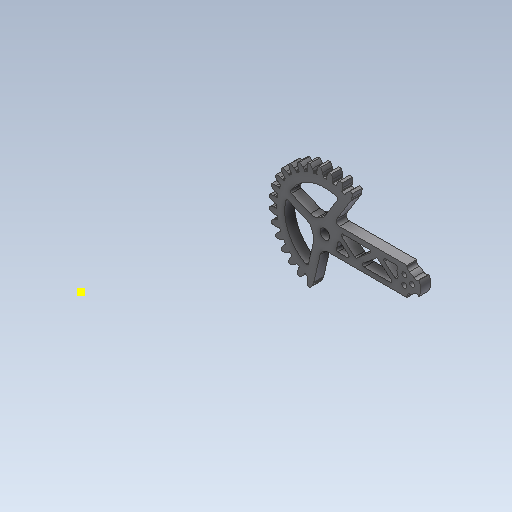
# Autodesk Inventor part: m2z32
Saved by Autodesk Inventor 2020 (Build 240168000, 168)
## iProperties
Created: 2020-01-07
Part Number: m2z32
Material: 一般
Document SubType Name: Modeling
Designer: hamaa
Density: 1 g/cm^3
Appearance: 既定
Mass: 10.1861 g
Surface Area: 77.3348 cm^2
Volume: 10.1861 cm^3
Author: hamaa
Autodesk Inventor part; units mm, degrees
(part 1 of 3)
ref_plane "YZ Plane" through (0, 0, 0) normal (1, 0, 0) x (0, 1, 0)
ref_plane "XZ Plane" through (0, 0, 0) normal (0, 1, 0) x (-1, 0, 0)
ref_plane "XY Plane" through (0, 0, 0) normal (0, 0, 1) x (1, 0, 0)
sketch "スケッチ1" plane through (0, 0, 0) normal (0, 0, 1) x (1, 0, 0)
  arc A0 (149.5779, 135.4165) -> (149.5278, 135.0527) centre (152.2771, 134.8591) ccw
  arc A1 (149.9451, 136.6514) -> (149.5779, 135.4165) centre (156.9811, 133.8877) ccw
  arc A2 (151.0923, 138.9012) -> (149.9451, 136.6514) centre (162.0444, 131.8989) ccw
  arc A3 (143.6233, 135.0423) -> (143.6451, 134.6758) centre (146.3794, 135.0222) ccw
  arc A4 (143.7424, 136.3252) -> (143.6233, 135.0423) centre (151.1825, 134.9872) ccw
  arc A5 (144.4287, 138.7555) -> (143.7424, 136.3252) centre (156.5365, 134.0244) ccw
  arc A6 (137.8561, 133.5137) -> (137.949, 133.1584) centre (140.5631, 134.0317) ccw
  arc A7 (137.7227, 134.7951) -> (137.8561, 133.5137) centre (145.2808, 134.9344) ccw
  arc A8 (137.9216, 137.3127) -> (137.7227, 134.7951) centre (150.7197, 135.0346) ccw
  arc A9 (132.4979, 130.8893) -> (132.6583, 130.559) centre (135.0518, 131.9254) ccw
  arc A10 (132.117, 132.1201) -> (132.4979, 130.8893) centre (139.5027, 133.7312) ccw
  arc A11 (131.821, 134.6281) -> (132.117, 132.1201) centre (144.8176, 134.8905) ccw
  arc A12 (127.7546, 127.27) -> (127.9764, 126.9773) centre (130.0574, 128.7845) ccw
  arc A13 (127.141, 128.4028) -> (127.7546, 127.27) centre (134.0705, 131.4238) ccw
  arc A14 (126.3614, 130.8049) -> (127.141, 128.4028) centre (139.0571, 133.5978) ccw
  arc A15 (123.8086, 122.7949) -> (124.0832, 122.5511) centre (125.7717, 124.7295) ccw
  arc A16 (122.9858, 123.7862) -> (123.8086, 122.7949) centre (129.1927, 128.1011) ccw
  arc A17 (121.7525, 125.99) -> (122.9858, 123.7862) centre (133.6594, 131.2061) ccw
  arc A18 (120.8115, 117.6359) -> (121.1284, 117.4504) centre (122.3594, 119.9163) ccw
  arc A19 (119.811, 118.4477) -> (120.8115, 117.6359) centre (125.057, 123.8905) ccw
  arc A20 (118.1715, 120.3685) -> (119.811, 118.4477) centre (128.832, 127.8073) ccw
  arc A21 (118.8784, 111.9914) -> (119.2254, 111.8712) centre (119.9517, 114.5299) ccw
  arc A22 (117.7388, 112.5923) -> (118.8784, 111.9914) centre (121.8221, 118.9541) ccw
  arc A23 (115.7561, 114.1565) -> (117.7388, 112.5923) centre (124.7605, 123.5321) ccw
  arc A24 (118.0837, 106.0781) -> (118.4474, 106.028) centre (118.641, 108.7773) ccw
  arc A25 (116.8487, 106.4453) -> (118.0837, 106.0781) centre (119.6124, 113.4813) ccw
  arc A26 (114.5989, 107.5925) -> (116.8487, 106.4453) centre (121.6012, 118.5446) ccw
  arc A27 (118.4578, 100.1235) -> (118.8243, 100.1453) centre (118.4779, 102.8796) ccw
  arc A28 (117.175, 100.2426) -> (118.4578, 100.1235) centre (118.5129, 107.6827) ccw
  arc A29 (114.7446, 100.9289) -> (117.175, 100.2426) centre (119.4757, 113.0367) ccw
  arc A30 (119.9864, 94.3563) -> (120.3417, 94.4491) centre (119.4685, 97.0633) ccw
  arc A31 (118.705, 94.2229) -> (119.9864, 94.3563) centre (118.5657, 101.781) ccw
  arc A32 (116.1874, 94.4218) -> (118.705, 94.2229) centre (118.4655, 107.2199) ccw
  arc A33 (122.6108, 88.9981) -> (122.9411, 89.1585) centre (121.5747, 91.552) ccw
  arc A34 (121.3801, 88.6172) -> (122.6108, 88.9981) centre (119.769, 96.0029) ccw
  arc A35 (118.8721, 88.3212) -> (121.3801, 88.6172) centre (118.6096, 101.3178) ccw
  arc A36 (126.2301, 84.2548) -> (126.5228, 84.4766) centre (124.7157, 86.5576) ccw
  arc A37 (125.0973, 83.6412) -> (126.2301, 84.2548) centre (122.0763, 90.5707) ccw
  arc A38 (122.6952, 82.8616) -> (125.0973, 83.6412) centre (119.9023, 95.5573) ccw
  arc A39 (130.7053, 80.3088) -> (130.949, 80.5834) centre (128.7706, 82.2718) ccw
  arc A40 (129.7139, 79.486) -> (130.7053, 80.3088) centre (125.3991, 85.6929) ccw
  arc A41 (127.5101, 78.2527) -> (129.7139, 79.486) centre (122.294, 90.1596) ccw
  arc A42 (135.8642, 77.3117) -> (136.0497, 77.6286) centre (133.5838, 78.8596) ccw
  arc A43 (135.0525, 76.3112) -> (135.8642, 77.3117) centre (129.6096, 81.5572) ccw
  arc A44 (133.1316, 74.6717) -> (135.0525, 76.3112) centre (125.6928, 85.3322) ccw
  arc A45 (141.5088, 75.3786) -> (141.6289, 75.7256) centre (138.9702, 76.4519) ccw
  arc A46 (140.9078, 74.239) -> (141.5088, 75.3786) centre (134.5461, 78.3223) ccw
  arc A47 (139.3437, 72.2563) -> (140.9078, 74.239) centre (129.9681, 81.2607) ccw
  arc A48 (147.422, 74.5839) -> (147.4721, 74.9476) centre (144.7228, 75.1412) ccw
  arc A49 (147.0549, 73.3489) -> (147.422, 74.5839) centre (140.0188, 76.1126) ccw
  arc A50 (145.9076, 71.0991) -> (147.0549, 73.3489) centre (134.9555, 78.1014) ccw
  arc A51 (153.3766, 74.958) -> (153.3548, 75.3245) centre (150.6206, 74.9781) ccw
  arc A52 (153.2575, 73.6752) -> (153.3766, 74.958) centre (145.8174, 75.0131) ccw
  arc A53 (152.5712, 71.2448) -> (153.2575, 73.6752) centre (140.4634, 75.9759) ccw
  arc A54 (159.1439, 76.4866) -> (159.051, 76.8419) centre (156.4368, 75.9687) ccw
  arc A55 (159.2773, 75.2052) -> (159.1439, 76.4866) centre (151.7192, 75.0659) ccw
  arc A56 (159.0783, 72.6876) -> (159.2773, 75.2052) centre (146.2802, 74.9657) ccw
  arc A57 (164.502, 79.111) -> (164.3416, 79.4413) centre (161.9481, 78.0749) ccw
  arc A58 (164.8829, 77.8803) -> (164.502, 79.111) centre (157.4972, 76.2692) ccw
  arc A59 (165.1789, 75.3722) -> (164.8829, 77.8803) centre (152.1823, 75.1098) ccw
  arc A60 (169.2453, 82.7303) -> (169.0235, 83.023) centre (166.9426, 81.2159) ccw
  arc A61 (169.8589, 81.5975) -> (169.2453, 82.7303) centre (162.9294, 78.5765) ccw
  arc A62 (170.6385, 79.1954) -> (169.8589, 81.5975) centre (157.9429, 76.4025) ccw
  arc A63 (173.1913, 87.2055) -> (172.9167, 87.4492) centre (171.2283, 85.2708) ccw
  arc A64 (174.0142, 86.2141) -> (173.1913, 87.2055) centre (167.8072, 81.8993) ccw
  arc A65 (175.2474, 84.0103) -> (174.0142, 86.2141) centre (163.3405, 78.7942) ccw
  arc A66 (176.1884, 92.3644) -> (175.8716, 92.5499) centre (174.6406, 90.084) ccw
  arc A67 (177.1889, 91.5526) -> (176.1884, 92.3644) centre (171.943, 86.1098) ccw
  arc A68 (178.8284, 89.6318) -> (177.1889, 91.5526) centre (168.1679, 82.193) ccw
  arc A69 (178.1215, 98.009) -> (177.7745, 98.1291) centre (177.0483, 95.4704) ccw
  arc A70 (179.2611, 97.408) -> (178.1215, 98.009) centre (175.1778, 91.0463) ccw
  arc A71 (181.2438, 95.8439) -> (179.2611, 97.408) centre (172.2395, 86.4683) ccw
  arc A72 (178.9163, 103.9222) -> (178.5525, 103.9723) centre (178.3589, 101.223) ccw
  arc A73 (180.1512, 103.5551) -> (178.9163, 103.9222) centre (177.3875, 96.519) ccw
  arc A74 (182.401, 102.4078) -> (180.1512, 103.5551) centre (175.3987, 91.4557) ccw
  arc A75 (178.5421, 109.8768) -> (178.1756, 109.855) centre (178.522, 107.1208) ccw
  arc A76 (179.825, 109.7577) -> (178.5421, 109.8768) centre (178.487, 102.3176) ccw
  arc A77 (182.2553, 109.0714) -> (179.825, 109.7577) centre (177.5242, 96.9636) ccw
  arc A78 (177.0135, 115.644) -> (176.6582, 115.5512) centre (177.5315, 112.937) ccw
  arc A79 (178.2949, 115.7775) -> (177.0135, 115.644) centre (178.4342, 108.2194) ccw
  arc A80 (180.8125, 115.5785) -> (178.2949, 115.7775) centre (178.5344, 102.7804) ccw
  arc A81 (174.3891, 121.0022) -> (174.0588, 120.8418) centre (175.4252, 118.4483) ccw
  arc A82 (175.6199, 121.3831) -> (174.3891, 121.0022) centre (177.231, 113.9974) ccw
  arc A83 (178.1279, 121.6791) -> (175.6199, 121.3831) centre (178.3903, 108.6825) ccw
  arc A84 (170.7698, 125.7455) -> (170.4771, 125.5237) centre (172.2843, 123.4427) ccw
  arc A85 (171.9026, 126.3591) -> (170.7698, 125.7455) centre (174.9236, 119.4296) ccw
  arc A86 (174.3047, 127.1387) -> (171.9026, 126.3591) centre (177.0976, 114.4431) ccw
  arc A87 (166.2947, 129.6915) -> (166.0509, 129.4169) centre (168.2293, 127.7285) ccw
  arc A88 (167.286, 130.5144) -> (166.2947, 129.6915) centre (171.6009, 124.3074) ccw
  arc A89 (169.4898, 131.7476) -> (167.286, 130.5144) centre (174.7059, 119.8407) ccw
  arc A90 (161.1357, 132.6886) -> (160.9502, 132.3718) centre (163.4161, 131.1408) ccw
  arc A91 (161.9475, 133.6891) -> (161.1357, 132.6886) centre (167.3903, 128.4432) ccw
  arc A92 (163.8683, 135.3286) -> (161.9475, 133.6891) centre (171.3071, 124.6681) ccw
  arc A93 (155.4912, 134.6217) -> (155.371, 134.2747) centre (158.0297, 133.5485) ccw
  arc A94 (156.0922, 135.7613) -> (155.4912, 134.6217) centre (162.4539, 131.678) ccw
  arc A95 (157.6563, 137.744) -> (156.0922, 135.7613) centre (167.0319, 128.7396) ccw
  arc A96 (147.4721, 135.0527) -> (147.422, 135.4165) centre (144.7228, 134.8591) ccw
  arc A97 (147.422, 135.4165) -> (147.0549, 136.6514) centre (140.0188, 133.8877) ccw
  arc A98 (147.0549, 136.6514) -> (145.9076, 138.9012) centre (134.9555, 131.8989) ccw
  arc A99 (141.6289, 134.2747) -> (141.5088, 134.6217) centre (138.9702, 133.5485) ccw
  arc A100 (141.5088, 134.6217) -> (140.9078, 135.7613) centre (134.5461, 131.678) ccw
  arc A101 (140.9078, 135.7613) -> (139.3437, 137.744) centre (129.9681, 128.7396) ccw
  arc A102 (136.0497, 132.3718) -> (135.8642, 132.6886) centre (133.5838, 131.1408) ccw
  arc A103 (135.8642, 132.6886) -> (135.0525, 133.6891) centre (129.6096, 128.4432) ccw
  arc A104 (135.0525, 133.6891) -> (133.1316, 135.3286) centre (125.6928, 124.6681) ccw
  arc A105 (130.949, 129.4169) -> (130.7053, 129.6915) centre (128.7706, 127.7285) ccw
  arc A106 (130.7053, 129.6915) -> (129.7139, 130.5144) centre (125.3991, 124.3074) ccw
  arc A107 (129.7139, 130.5144) -> (127.5101, 131.7476) centre (122.294, 119.8407) ccw
  arc A108 (126.5228, 125.5237) -> (126.2301, 125.7455) centre (124.7157, 123.4427) ccw
  arc A109 (126.2301, 125.7455) -> (125.0973, 126.3591) centre (122.0763, 119.4296) ccw
  arc A110 (125.0973, 126.3591) -> (122.6952, 127.1387) centre (119.9023, 114.4431) ccw
  arc A111 (122.9411, 120.8418) -> (122.6108, 121.0022) centre (121.5747, 118.4483) ccw
  arc A112 (122.6108, 121.0022) -> (121.3801, 121.3831) centre (119.769, 113.9974) ccw
  arc A113 (121.3801, 121.3831) -> (118.8721, 121.6791) centre (118.6096, 108.6825) ccw
  arc A114 (120.3417, 115.5512) -> (119.9864, 115.644) centre (119.4685, 112.937) ccw
  arc A115 (119.9864, 115.644) -> (118.705, 115.7775) centre (118.5657, 108.2194) ccw
  arc A116 (118.705, 115.7775) -> (116.1874, 115.5785) centre (118.4655, 102.7804) ccw
  arc A117 (118.8243, 109.855) -> (118.4578, 109.8768) centre (118.4779, 107.1208) ccw
  arc A118 (118.4578, 109.8768) -> (117.175, 109.7577) centre (118.5129, 102.3176) ccw
  arc A119 (117.175, 109.7577) -> (114.7446, 109.0714) centre (119.4757, 96.9636) ccw
  arc A120 (118.4474, 103.9723) -> (118.0837, 103.9222) centre (118.641, 101.223) ccw
  arc A121 (118.0837, 103.9222) -> (116.8487, 103.5551) centre (119.6124, 96.519) ccw
  arc A122 (116.8487, 103.5551) -> (114.5989, 102.4078) centre (121.6012, 91.4557) ccw
  arc A123 (119.2254, 98.1291) -> (118.8784, 98.009) centre (119.9517, 95.4704) ccw
  arc A124 (118.8784, 98.009) -> (117.7388, 97.408) centre (121.8221, 91.0463) ccw
  arc A125 (117.7388, 97.408) -> (115.7561, 95.8439) centre (124.7605, 86.4683) ccw
  arc A126 (121.1284, 92.5499) -> (120.8115, 92.3644) centre (122.3594, 90.084) ccw
  arc A127 (120.8115, 92.3644) -> (119.811, 91.5526) centre (125.057, 86.1098) ccw
  arc A128 (119.811, 91.5526) -> (118.1715, 89.6318) centre (128.832, 82.193) ccw
  arc A129 (124.0832, 87.4492) -> (123.8086, 87.2055) centre (125.7717, 85.2708) ccw
  arc A130 (123.8086, 87.2055) -> (122.9858, 86.2141) centre (129.1927, 81.8993) ccw
  arc A131 (122.9858, 86.2141) -> (121.7525, 84.0103) centre (133.6594, 78.7942) ccw
  arc A132 (127.9764, 83.023) -> (127.7546, 82.7303) centre (130.0574, 81.2159) ccw
  arc A133 (127.7546, 82.7303) -> (127.141, 81.5975) centre (134.0705, 78.5765) ccw
  arc A134 (127.141, 81.5975) -> (126.3614, 79.1954) centre (139.0571, 76.4025) ccw
  arc A135 (132.6583, 79.4413) -> (132.4979, 79.111) centre (135.0518, 78.0749) ccw
  arc A136 (132.4979, 79.111) -> (132.117, 77.8803) centre (139.5027, 76.2692) ccw
  arc A137 (132.117, 77.8803) -> (131.821, 75.3722) centre (144.8176, 75.1098) ccw
  arc A138 (137.949, 76.8419) -> (137.8561, 76.4866) centre (140.5631, 75.9687) ccw
  arc A139 (137.8561, 76.4866) -> (137.7227, 75.2052) centre (145.2808, 75.0659) ccw
  arc A140 (137.7227, 75.2052) -> (137.9216, 72.6876) centre (150.7197, 74.9657) ccw
  arc A141 (143.6451, 75.3245) -> (143.6233, 74.958) centre (146.3794, 74.9781) ccw
  arc A142 (143.6233, 74.958) -> (143.7424, 73.6752) centre (151.1825, 75.0131) ccw
  arc A143 (143.7424, 73.6752) -> (144.4287, 71.2448) centre (156.5365, 75.9759) ccw
  arc A144 (149.5278, 74.9476) -> (149.5779, 74.5839) centre (152.2771, 75.1412) ccw
  arc A145 (149.5779, 74.5839) -> (149.9451, 73.3489) centre (156.9811, 76.1126) ccw
  arc A146 (149.9451, 73.3489) -> (151.0923, 71.0991) centre (162.0444, 78.1014) ccw
  arc A147 (155.371, 75.7256) -> (155.4912, 75.3786) centre (158.0297, 76.4519) ccw
  arc A148 (155.4912, 75.3786) -> (156.0922, 74.239) centre (162.4539, 78.3223) ccw
  arc A149 (156.0922, 74.239) -> (157.6563, 72.2563) centre (167.0319, 81.2607) ccw
  arc A150 (160.9502, 77.6286) -> (161.1357, 77.3117) centre (163.4161, 78.8596) ccw
  arc A151 (161.1357, 77.3117) -> (161.9475, 76.3112) centre (167.3903, 81.5572) ccw
  arc A152 (161.9475, 76.3112) -> (163.8683, 74.6717) centre (171.3071, 85.3322) ccw
  arc A153 (166.0509, 80.5834) -> (166.2947, 80.3088) centre (168.2293, 82.2718) ccw
  arc A154 (166.2947, 80.3088) -> (167.286, 79.486) centre (171.6009, 85.6929) ccw
  arc A155 (167.286, 79.486) -> (169.4898, 78.2527) centre (174.7059, 90.1596) ccw
  arc A156 (170.4771, 84.4766) -> (170.7698, 84.2548) centre (172.2843, 86.5576) ccw
  arc A157 (170.7698, 84.2548) -> (171.9026, 83.6412) centre (174.9236, 90.5707) ccw
  arc A158 (171.9026, 83.6412) -> (174.3047, 82.8616) centre (177.0976, 95.5573) ccw
  arc A159 (174.0588, 89.1585) -> (174.3891, 88.9981) centre (175.4252, 91.552) ccw
  arc A160 (174.3891, 88.9981) -> (175.6199, 88.6172) centre (177.231, 96.0029) ccw
  arc A161 (175.6199, 88.6172) -> (178.1279, 88.3212) centre (178.3903, 101.3178) ccw
  arc A162 (176.6582, 94.4491) -> (177.0135, 94.3563) centre (177.5315, 97.0633) ccw
  arc A163 (177.0135, 94.3563) -> (178.2949, 94.2229) centre (178.4342, 101.781) ccw
  arc A164 (178.2949, 94.2229) -> (180.8125, 94.4218) centre (178.5344, 107.2199) ccw
  arc A165 (178.1756, 100.1453) -> (178.5421, 100.1235) centre (178.522, 102.8796) ccw
  arc A166 (178.5421, 100.1235) -> (179.825, 100.2426) centre (178.487, 107.6827) ccw
  arc A167 (179.825, 100.2426) -> (182.2553, 100.9289) centre (177.5242, 113.0367) ccw
  arc A168 (178.5525, 106.028) -> (178.9163, 106.0781) centre (178.3589, 108.7773) ccw
  arc A169 (178.9163, 106.0781) -> (180.1512, 106.4453) centre (177.3875, 113.4813) ccw
  arc A170 (180.1512, 106.4453) -> (182.401, 107.5925) centre (175.3987, 118.5446) ccw
  arc A171 (177.7745, 111.8712) -> (178.1215, 111.9914) centre (177.0483, 114.5299) ccw
  arc A172 (178.1215, 111.9914) -> (179.2611, 112.5923) centre (175.1778, 118.9541) ccw
  arc A173 (179.2611, 112.5923) -> (181.2438, 114.1565) centre (172.2395, 123.5321) ccw
  arc A174 (175.8716, 117.4504) -> (176.1884, 117.6359) centre (174.6406, 119.9163) ccw
  arc A175 (176.1884, 117.6359) -> (177.1889, 118.4477) centre (171.943, 123.8905) ccw
  arc A176 (177.1889, 118.4477) -> (178.8284, 120.3685) centre (168.1679, 127.8073) ccw
  arc A177 (172.9167, 122.5511) -> (173.1913, 122.7949) centre (171.2283, 124.7295) ccw
  arc A178 (173.1913, 122.7949) -> (174.0142, 123.7862) centre (167.8072, 128.1011) ccw
  arc A179 (174.0142, 123.7862) -> (175.2474, 125.99) centre (163.3405, 131.2061) ccw
  arc A180 (169.0235, 126.9773) -> (169.2453, 127.27) centre (166.9426, 128.7845) ccw
  arc A181 (169.2453, 127.27) -> (169.8589, 128.4028) centre (162.9294, 131.4238) ccw
  arc A182 (169.8589, 128.4028) -> (170.6385, 130.8049) centre (157.9429, 133.5978) ccw
  arc A183 (164.3416, 130.559) -> (164.502, 130.8893) centre (161.9481, 131.9254) ccw
  arc A184 (164.502, 130.8893) -> (164.8829, 132.1201) centre (157.4972, 133.7312) ccw
  arc A185 (164.8829, 132.1201) -> (165.1789, 134.6281) centre (152.1823, 134.8905) ccw
  arc A186 (159.051, 133.1584) -> (159.1439, 133.5137) centre (156.4368, 134.0317) ccw
  arc A187 (159.1439, 133.5137) -> (159.2773, 134.7951) centre (151.7192, 134.9344) ccw
  arc A188 (159.2773, 134.7951) -> (159.0783, 137.3127) centre (146.2802, 135.0346) ccw
  arc A189 (153.3548, 134.6758) -> (153.3766, 135.0423) centre (150.6206, 135.0222) ccw
  arc A190 (153.3766, 135.0423) -> (153.2575, 136.3252) centre (145.8174, 134.9872) ccw
  arc A191 (153.2575, 136.3252) -> (152.5712, 138.7555) centre (140.4634, 134.0244) ccw
  arc A192 (149.5083, 134.4829) -> (147.4916, 134.4829) centre (148.5, 105.0002) ccw
  arc A193 (143.7371, 134.1131) -> (141.7592, 133.7197) centre (148.5, 105.0002) ccw
  arc A194 (138.149, 132.6246) -> (136.2858, 131.8528) centre (148.5, 105.0002) ccw
  arc A195 (132.9586, 130.0744) -> (131.2818, 128.954) centre (148.5, 105.0002) ccw
  arc A196 (128.3655, 126.5606) -> (126.9395, 125.1346) centre (148.5, 105.0002) ccw
  arc A197 (124.5462, 122.2183) -> (123.4257, 120.5415) centre (148.5, 105.0002) ccw
  arc A198 (121.6473, 117.2143) -> (120.8756, 115.3511) centre (148.5, 105.0002) ccw
  arc A199 (119.7804, 111.7409) -> (119.387, 109.763) centre (148.5, 105.0002) ccw
  arc A200 (119.0172, 106.0085) -> (119.0172, 103.9918) centre (148.5, 105.0002) ccw
  arc A201 (119.387, 100.2373) -> (119.7804, 98.2594) centre (148.5, 105.0002) ccw
  arc A202 (120.8756, 94.6492) -> (121.6473, 92.786) centre (148.5, 105.0002) ccw
  arc A203 (123.4257, 89.4588) -> (124.5462, 87.782) centre (148.5, 105.0002) ccw
  arc A204 (126.9395, 84.8657) -> (128.3655, 83.4397) centre (148.5, 105.0002) ccw
  arc A205 (131.2818, 81.0464) -> (132.9586, 79.9259) centre (148.5, 105.0002) ccw
  arc A206 (136.2858, 78.1475) -> (138.149, 77.3758) centre (148.5, 105.0002) ccw
  arc A207 (141.7592, 76.2806) -> (143.7371, 75.8872) centre (148.5, 105.0002) ccw
  arc A208 (147.4916, 75.5174) -> (149.5083, 75.5174) centre (148.5, 105.0002) ccw
  arc A209 (153.2628, 75.8872) -> (155.2407, 76.2806) centre (148.5, 105.0002) ccw
  arc A210 (158.8509, 77.3758) -> (160.7141, 78.1475) centre (148.5, 105.0002) ccw
  arc A211 (164.0413, 79.9259) -> (165.7181, 81.0464) centre (148.5, 105.0002) ccw
  arc A212 (168.6344, 83.4397) -> (170.0604, 84.8657) centre (148.5, 105.0002) ccw
  arc A213 (172.4538, 87.782) -> (173.5742, 89.4588) centre (148.5, 105.0002) ccw
  arc A214 (175.3526, 92.786) -> (176.1244, 94.6492) centre (148.5, 105.0002) ccw
  arc A215 (177.2195, 98.2594) -> (177.6129, 100.2373) centre (148.5, 105.0002) ccw
  arc A216 (177.9827, 103.9918) -> (177.9827, 106.0085) centre (148.5, 105.0002) ccw
  arc A217 (177.6129, 109.763) -> (177.2195, 111.7409) centre (148.5, 105.0002) ccw
  arc A218 (176.1244, 115.3511) -> (175.3526, 117.2143) centre (148.5, 105.0002) ccw
  arc A219 (173.5742, 120.5415) -> (172.4538, 122.2183) centre (148.5, 105.0002) ccw
  arc A220 (170.0604, 125.1346) -> (168.6344, 126.5606) centre (148.5, 105.0002) ccw
  arc A221 (165.7181, 128.954) -> (164.0413, 130.0744) centre (148.5, 105.0002) ccw
  arc A222 (160.7141, 131.8528) -> (158.8509, 132.6246) centre (148.5, 105.0002) ccw
  arc A223 (155.2407, 133.7197) -> (153.2628, 134.1131) centre (148.5, 105.0002) ccw
  arc A224 (145.9076, 138.9012) -> (144.4287, 138.7555) centre (148.5, 105.0002) ccw
  arc A225 (139.3437, 137.744) -> (137.9216, 137.3127) centre (148.5, 105.0002) ccw
  arc A226 (133.1316, 135.3286) -> (131.821, 134.6281) centre (148.5, 105.0002) ccw
  arc A227 (127.5101, 131.7476) -> (126.3614, 130.8049) centre (148.5, 105.0002) ccw
  arc A228 (122.6952, 127.1387) -> (121.7525, 125.99) centre (148.5, 105.0002) ccw
  arc A229 (118.8721, 121.6791) -> (118.1715, 120.3685) centre (148.5, 105.0002) ccw
  arc A230 (116.1874, 115.5785) -> (115.7561, 114.1565) centre (148.5, 105.0002) ccw
  arc A231 (114.7446, 109.0714) -> (114.5989, 107.5925) centre (148.5, 105.0002) ccw
  arc A232 (114.5989, 102.4078) -> (114.7446, 100.9289) centre (148.5, 105.0002) ccw
  arc A233 (115.7561, 95.8439) -> (116.1874, 94.4218) centre (148.5, 105.0002) ccw
  arc A234 (118.1715, 89.6318) -> (118.8721, 88.3212) centre (148.5, 105.0002) ccw
  arc A235 (121.7525, 84.0103) -> (122.6952, 82.8616) centre (148.5, 105.0002) ccw
  arc A236 (126.3614, 79.1954) -> (127.5101, 78.2527) centre (148.5, 105.0002) ccw
  arc A237 (131.821, 75.3722) -> (133.1316, 74.6717) centre (148.5, 105.0002) ccw
  arc A238 (137.9216, 72.6876) -> (139.3437, 72.2563) centre (148.5, 105.0002) ccw
  arc A239 (144.4287, 71.2448) -> (145.9076, 71.0991) centre (148.5, 105.0002) ccw
  arc A240 (151.0923, 71.0991) -> (152.5712, 71.2448) centre (148.5, 105.0002) ccw
  arc A241 (157.6563, 72.2563) -> (159.0783, 72.6876) centre (148.5, 105.0002) ccw
  arc A242 (163.8683, 74.6717) -> (165.1789, 75.3722) centre (148.5, 105.0002) ccw
  arc A243 (169.4898, 78.2527) -> (170.6385, 79.1954) centre (148.5, 105.0002) ccw
  arc A244 (174.3047, 82.8616) -> (175.2474, 84.0103) centre (148.5, 105.0002) ccw
  arc A245 (178.1279, 88.3212) -> (178.8284, 89.6318) centre (148.5, 105.0002) ccw
  arc A246 (180.8125, 94.4218) -> (181.2438, 95.8439) centre (148.5, 105.0002) ccw
  arc A247 (182.2553, 100.9289) -> (182.401, 102.4078) centre (148.5, 105.0002) ccw
  arc A248 (182.401, 107.5925) -> (182.2553, 109.0714) centre (148.5, 105.0002) ccw
  arc A249 (181.2438, 114.1565) -> (180.8125, 115.5785) centre (148.5, 105.0002) ccw
  arc A250 (178.8284, 120.3685) -> (178.1279, 121.6791) centre (148.5, 105.0002) ccw
  arc A251 (175.2474, 125.99) -> (174.3047, 127.1387) centre (148.5, 105.0002) ccw
  arc A252 (170.6385, 130.8049) -> (169.4898, 131.7476) centre (148.5, 105.0002) ccw
  arc A253 (165.1789, 134.6281) -> (163.8683, 135.3286) centre (148.5, 105.0002) ccw
  arc A254 (159.0783, 137.3127) -> (157.6563, 137.744) centre (148.5, 105.0002) ccw
  arc A255 (152.5712, 138.7555) -> (151.0923, 138.9012) centre (148.5, 105.0002) ccw
  line L0 (149.5083, 134.4829) -> (149.5278, 135.0527)
  line L1 (143.7371, 134.1131) -> (143.6451, 134.6758)
  line L2 (138.149, 132.6246) -> (137.949, 133.1584)
  line L3 (132.9586, 130.0744) -> (132.6583, 130.559)
  line L4 (128.3655, 126.5606) -> (127.9764, 126.9773)
  line L5 (124.5462, 122.2183) -> (124.0832, 122.5511)
  line L6 (121.6473, 117.2143) -> (121.1284, 117.4504)
  line L7 (119.7804, 111.7409) -> (119.2254, 111.8712)
  line L8 (119.0172, 106.0085) -> (118.4474, 106.028)
  line L9 (119.387, 100.2373) -> (118.8243, 100.1453)
  line L10 (120.8756, 94.6492) -> (120.3417, 94.4491)
  line L11 (123.4257, 89.4588) -> (122.9411, 89.1585)
  line L12 (126.9395, 84.8657) -> (126.5228, 84.4766)
  line L13 (131.2818, 81.0464) -> (130.949, 80.5834)
  line L14 (136.2858, 78.1475) -> (136.0497, 77.6286)
  line L15 (141.7592, 76.2806) -> (141.6289, 75.7256)
  line L16 (147.4916, 75.5174) -> (147.4721, 74.9476)
  line L17 (153.2628, 75.8872) -> (153.3548, 75.3245)
  line L18 (158.8509, 77.3758) -> (159.051, 76.8419)
  line L19 (164.0413, 79.9259) -> (164.3416, 79.4413)
  line L20 (168.6344, 83.4397) -> (169.0235, 83.023)
  line L21 (172.4538, 87.782) -> (172.9167, 87.4492)
  line L22 (175.3526, 92.786) -> (175.8716, 92.5499)
  line L23 (177.2195, 98.2594) -> (177.7745, 98.1291)
  line L24 (177.9827, 103.9918) -> (178.5525, 103.9723)
  line L25 (177.6129, 109.763) -> (178.1756, 109.855)
  line L26 (176.1244, 115.3511) -> (176.6582, 115.5512)
  line L27 (173.5742, 120.5415) -> (174.0588, 120.8418)
  line L28 (170.0604, 125.1346) -> (170.4771, 125.5237)
  line L29 (165.7181, 128.954) -> (166.0509, 129.4169)
  line L30 (160.7141, 131.8528) -> (160.9502, 132.3718)
  line L31 (155.2407, 133.7197) -> (155.371, 134.2747)
  line L32 (147.4916, 134.4829) -> (147.4721, 135.0527)
  line L33 (141.7592, 133.7197) -> (141.6289, 134.2747)
  line L34 (136.2858, 131.8528) -> (136.0497, 132.3718)
  line L35 (131.2818, 128.954) -> (130.949, 129.4169)
  line L36 (126.9395, 125.1346) -> (126.5228, 125.5237)
  line L37 (123.4257, 120.5415) -> (122.9411, 120.8418)
  line L38 (120.8756, 115.3511) -> (120.3417, 115.5512)
  line L39 (119.387, 109.763) -> (118.8243, 109.855)
  line L40 (119.0172, 103.9918) -> (118.4474, 103.9723)
  line L41 (119.7804, 98.2594) -> (119.2254, 98.1291)
  line L42 (121.6473, 92.786) -> (121.1284, 92.5499)
  line L43 (124.5462, 87.782) -> (124.0832, 87.4492)
  line L44 (128.3655, 83.4397) -> (127.9764, 83.023)
  line L45 (132.9586, 79.9259) -> (132.6583, 79.4413)
  line L46 (138.149, 77.3758) -> (137.949, 76.8419)
  line L47 (143.7371, 75.8872) -> (143.6451, 75.3245)
  line L48 (149.5083, 75.5174) -> (149.5278, 74.9476)
  line L49 (155.2407, 76.2806) -> (155.371, 75.7256)
  line L50 (160.7141, 78.1475) -> (160.9502, 77.6286)
  line L51 (165.7181, 81.0464) -> (166.0509, 80.5834)
  line L52 (170.0604, 84.8657) -> (170.4771, 84.4766)
  line L53 (173.5742, 89.4588) -> (174.0588, 89.1585)
  line L54 (176.1244, 94.6492) -> (176.6582, 94.4491)
  line L55 (177.6129, 100.2373) -> (178.1756, 100.1453)
  line L56 (177.9827, 106.0085) -> (178.5525, 106.028)
  line L57 (177.2195, 111.7409) -> (177.7745, 111.8712)
  line L58 (175.3526, 117.2143) -> (175.8716, 117.4504)
  line L59 (172.4538, 122.2183) -> (172.9167, 122.5511)
  line L60 (168.6344, 126.5606) -> (169.0235, 126.9773)
  line L61 (164.0413, 130.0744) -> (164.3416, 130.559)
  line L62 (158.8509, 132.6246) -> (159.051, 133.1584)
  line L63 (153.2628, 134.1131) -> (153.3548, 134.6758)
  line L64 (112.5, 105) -> (184.5, 105)
  line L65 (148.5, 69) -> (148.5, 141)
  line L66 (202.5, 139.0002) -> (272.5, 139.0002)
  line L67 (202.5, 131.0002) -> (272.5, 131.0002)
  line L68 (202.5, 123.0002) -> (272.5, 123.0002)
  line L69 (202.5, 115.0002) -> (272.5, 115.0002)
  line L70 (202.5, 107.0002) -> (272.5, 107.0002)
  line L71 (202.5, 99.0002) -> (272.5, 99.0002)
  line L72 (202.5, 91.0002) -> (272.5, 91.0002)
  line L73 (202.5, 83.0002) -> (272.5, 83.0002)
  line L74 (202.5, 75.0002) -> (272.5, 75.0002)
  line L75 (202.5, 67.0002) -> (272.5, 67.0002)
  line L76 (202.5, 59.0002) -> (272.5, 59.0002)
  line L77 (202.5, 51.0002) -> (272.5, 51.0002)
  line L78 (202.5, 43.0002) -> (272.5, 43.0002)
  line L79 (202.5, 139.0002) -> (202.5, 43.0002)
  line L80 (272.5, 139.0002) -> (272.5, 43.0002)
  line L81 (237.5, 131.0002) -> (237.5, 43.0002)
  point P0 (0, 0)
  point P1 (208.5, 133)
  point P2 (211, 125)
  point P3 (211, 117)
  point P4 (208.5, 109)
  point P5 (211, 101)
  point P6 (206, 93)
  point P7 (208.5, 85)
  point P8 (208.5, 77)
  point P9 (208.5, 69)
  point P10 (211, 61)
  point P11 (211, 53)
  point P12 (208.5, 45)
  point P13 (238.5, 125)
  point P14 (253.5, 117)
  point P15 (254.75, 109)
  point P16 (251, 101)
  point P17 (253.5, 93)
  point P18 (247.25, 85)
  point P19 (253.5, 77)
  point P20 (253.5, 69)
  point P21 (248.5, 61)
  point P22 (256, 53)
  point P23 (256, 45)
  point P24 (149.5, 154.5)
  point P25 (149.5, 148.5)
  point P26 (166.75, 154.5)
  point P27 (167.8125, 148.5)
  constraints: 384 point on circle, 192 centre point, 189 equal radius, 160 end point, 128 tangent, 45 parallel, 34 horizontal, 18 perpendicular, 2 horizontal alignment, 2 midpoint, 2 vertical alignment, 243 other
extrude "押し出し1" add sketch "スケッチ1" along normal blind 6 contours A1 A2 A255 A191 A190 A189 L63 A223 L31 A93 A94 A95 A254 A188 A187 A186 L62 A222 L30 A90 A91 A92 A253 A185 A184 A183 L61 A221 L29 A87 A88 A89 A252 A182 A181 A180 L60 A220 L28 A84 A85 A86 A251 A179 A178 A177 L59 A219 L27 A81 A82 A83 A250 A176 A175 A174 L58 A218 L26 A78 A79 A80 A249 A173 A172 A171 L57 A217 L25 A75 A76 A77 A248 A170 A169 A168 L56 A216 L64 L65 A192 L0 A0 | L65 L64 A200 L8 A24 A25 A26 A231 A119 A118 A117 L39 A199 L7 A21 A22 A23 A230 A116 A115 A114 L38 A198 L6 A18 A19 A20 A229 A113 A112 A111 L37 A197 L5 A15 A16 A17 A228 A110 A109 A108 L36 A196 L4 A12 A13 A14 A227 A107 A106 A105 L35 A195 L3 A9 A10 A11 A226 A104 A103 A102 L34 A194 L2 A6 A7 A8 A225 A101 A100 A99 L33 A193 L1 A3 A4 A5 A224 A98 A97 A96 L32 A192 | L65 A208 L16 A48 A49 A50 A239 A143 A142 A141 L47 A207 L15 A45 A46 A47 A238 A140 A139 A138 L46 A206 L14 A42 A43 A44 A237 A137 A136 A135 L45 A205 L13 A39 A40 A41 A236 A134 A133 A132 L44 A204 L12 A36 A37 A38 A235 A131 A130 A129 L43 A203 L11 A33 A34 A35 A234 A128 A127 A126 L42 A202 L10 A30 A31 A32 A233 A125 A124 A123 L41 A201 L9 A27 A28 A29 A232 A122 A121 A120 L40 A200 L64 | L64 A216 L24 A72 A73 A74 A247 A167 A166 A165 L55 A215 L23 A69 A70 A71 A246 A164 A163 A162 L54 A214 L22 A66 A67 A68 A245 A161 A160 A159 L53 A213 L21 A63 A64 A65 A244 A158 A157 A156 L52 A212 L20 A60 A61 A62 A243 A155 A154 A153 L51 A211 L19 A57 A58 A59 A242 A152 A151 A150 L50 A210 L18 A54 A55 A56 A241 A149 A148 A147 L49 A209 L17 A51 A52 A53 A240 A146 A145 A144 L48 A208 L65
sketch "スケッチ2" plane through (0, 0, 6) normal (0, 0, 1) x (1, 0, 0)
  arc A0 (161.1357, 132.6886) -> (160.9502, 132.3718) centre (163.4161, 131.1408) ccw projected
  line L0 (160.9502, 132.3718) -> (160.7141, 131.8528) projected
  arc A1 (160.7141, 131.8528) -> (158.8509, 132.6246) centre (148.5, 105.0002) ccw projected
  line L1 (158.8509, 132.6246) -> (159.051, 133.1584) projected
  arc A2 (159.051, 133.1584) -> (159.1439, 133.5137) centre (156.4368, 134.0317) ccw projected
  arc A3 (159.1439, 133.5137) -> (159.2773, 134.7951) centre (151.7192, 134.9344) ccw projected
  arc A4 (159.2773, 134.7951) -> (159.0783, 137.3127) centre (146.2802, 135.0346) ccw projected
  arc A5 (159.0783, 137.3127) -> (157.6563, 137.744) centre (148.5, 105.0002) ccw projected
  arc A6 (157.6563, 137.744) -> (156.0922, 135.7613) centre (167.0319, 128.7396) ccw projected
  arc A7 (156.0922, 135.7613) -> (155.4912, 134.6217) centre (162.4539, 131.678) ccw projected
  arc A8 (155.4912, 134.6217) -> (155.371, 134.2747) centre (158.0297, 133.5485) ccw projected
  line L2 (155.371, 134.2747) -> (155.2407, 133.7197) projected
  arc A9 (155.2407, 133.7197) -> (153.2628, 134.1131) centre (148.5, 105.0002) ccw projected
  line L3 (153.2628, 134.1131) -> (153.3548, 134.6758) projected
  arc A10 (153.3548, 134.6758) -> (153.3766, 135.0423) centre (150.6206, 135.0222) ccw projected
  arc A11 (153.3766, 135.0423) -> (153.2575, 136.3252) centre (145.8174, 134.9872) ccw projected
  arc A12 (153.2575, 136.3252) -> (152.5712, 138.7555) centre (140.4634, 134.0244) ccw projected
  arc A13 (152.5712, 138.7555) -> (151.0923, 138.9012) centre (148.5, 105.0002) ccw projected
  arc A14 (151.0923, 138.9012) -> (149.9451, 136.6514) centre (162.0444, 131.8989) ccw projected
  arc A15 (149.9451, 136.6514) -> (149.5779, 135.4165) centre (156.9811, 133.8877) ccw projected
  arc A16 (149.5779, 135.4165) -> (149.5278, 135.0527) centre (152.2771, 134.8591) ccw projected
  line L4 (149.5278, 135.0527) -> (149.5083, 134.4829) projected
  arc A17 (149.5083, 134.4829) -> (147.4916, 134.4829) centre (148.5, 105.0002) ccw projected
  line L5 (147.4916, 134.4829) -> (147.4721, 135.0527) projected
  arc A18 (147.4721, 135.0527) -> (147.422, 135.4165) centre (144.7228, 134.8591) ccw projected
  arc A19 (147.422, 135.4165) -> (147.0549, 136.6514) centre (140.0188, 133.8877) ccw projected
  arc A20 (147.0549, 136.6514) -> (145.9076, 138.9012) centre (134.9555, 131.8989) ccw projected
  arc A21 (145.9076, 138.9012) -> (144.4287, 138.7555) centre (148.5, 105.0002) ccw projected
  arc A22 (144.4287, 138.7555) -> (143.7424, 136.3252) centre (156.5365, 134.0244) ccw projected
  arc A23 (143.7424, 136.3252) -> (143.6233, 135.0423) centre (151.1825, 134.9872) ccw projected
  arc A24 (143.6233, 135.0423) -> (143.6451, 134.6758) centre (146.3794, 135.0222) ccw projected
  line L6 (143.6451, 134.6758) -> (143.7371, 134.1131) projected
  arc A25 (143.7371, 134.1131) -> (141.7592, 133.7197) centre (148.5, 105.0002) ccw projected
  line L7 (141.7592, 133.7197) -> (141.6289, 134.2747) projected
  arc A26 (141.6289, 134.2747) -> (141.5088, 134.6217) centre (138.9702, 133.5485) ccw projected
  arc A27 (141.5088, 134.6217) -> (140.9078, 135.7613) centre (134.5461, 131.678) ccw projected
  arc A28 (140.9078, 135.7613) -> (139.3437, 137.744) centre (129.9681, 128.7396) ccw projected
  arc A29 (139.3437, 137.744) -> (137.9216, 137.3127) centre (148.5, 105.0002) ccw projected
  arc A30 (137.9216, 137.3127) -> (137.7227, 134.7951) centre (150.7197, 135.0346) ccw projected
  arc A31 (137.7227, 134.7951) -> (137.8561, 133.5137) centre (145.2808, 134.9344) ccw projected
  arc A32 (137.8561, 133.5137) -> (137.949, 133.1584) centre (140.5631, 134.0317) ccw projected
  line L8 (137.949, 133.1584) -> (138.149, 132.6246) projected
  arc A33 (138.149, 132.6246) -> (136.2858, 131.8528) centre (148.5, 105.0002) ccw projected
  line L9 (136.2858, 131.8528) -> (136.0497, 132.3718) projected
  arc A34 (136.0497, 132.3718) -> (135.8642, 132.6886) centre (133.5838, 131.1408) ccw projected
  arc A35 (135.8642, 132.6886) -> (135.0525, 133.6891) centre (129.6096, 128.4432) ccw projected
  arc A36 (135.0525, 133.6891) -> (133.1316, 135.3286) centre (125.6928, 124.6681) ccw projected
  arc A37 (133.1316, 135.3286) -> (131.821, 134.6281) centre (148.5, 105.0002) ccw projected
  arc A38 (131.821, 134.6281) -> (132.117, 132.1201) centre (144.8176, 134.8905) ccw projected
  arc A39 (132.117, 132.1201) -> (132.4979, 130.8893) centre (139.5027, 133.7312) ccw projected
  arc A40 (132.4979, 130.8893) -> (132.6583, 130.559) centre (135.0518, 131.9254) ccw projected
  line L10 (132.6583, 130.559) -> (132.9586, 130.0744) projected
  arc A41 (132.9586, 130.0744) -> (131.2818, 128.954) centre (148.5, 105.0002) ccw projected
  line L11 (131.2818, 128.954) -> (130.949, 129.4169) projected
  arc A42 (130.949, 129.4169) -> (130.7053, 129.6915) centre (128.7706, 127.7285) ccw projected
  arc A43 (130.7053, 129.6915) -> (129.7139, 130.5144) centre (125.3991, 124.3074) ccw projected
  arc A44 (129.7139, 130.5144) -> (127.5101, 131.7476) centre (122.294, 119.8407) ccw projected
  arc A45 (127.5101, 131.7476) -> (126.3614, 130.8049) centre (148.5, 105.0002) ccw projected
  arc A46 (126.3614, 130.8049) -> (127.141, 128.4028) centre (139.0571, 133.5978) ccw projected
  arc A47 (127.141, 128.4028) -> (127.7546, 127.27) centre (134.0705, 131.4238) ccw projected
  arc A48 (127.7546, 127.27) -> (127.9764, 126.9773) centre (130.0574, 128.7845) ccw projected
  line L12 (127.9764, 126.9773) -> (128.3655, 126.5606) projected
  arc A49 (128.3655, 126.5606) -> (126.9395, 125.1346) centre (148.5, 105.0002) ccw projected
  line L13 (126.9395, 125.1346) -> (126.5228, 125.5237) projected
  arc A50 (126.5228, 125.5237) -> (126.2301, 125.7455) centre (124.7157, 123.4427) ccw projected
  arc A51 (126.2301, 125.7455) -> (125.0973, 126.3591) centre (122.0763, 119.4296) ccw projected
  arc A52 (125.0973, 126.3591) -> (122.6952, 127.1387) centre (119.9023, 114.4431) ccw projected
  arc A53 (122.6952, 127.1387) -> (121.7525, 125.99) centre (148.5, 105.0002) ccw projected
  arc A54 (121.7525, 125.99) -> (122.9858, 123.7862) centre (133.6594, 131.2061) ccw projected
  arc A55 (122.9858, 123.7862) -> (123.8086, 122.7949) centre (129.1927, 128.1011) ccw projected
  arc A56 (123.8086, 122.7949) -> (124.0832, 122.5511) centre (125.7717, 124.7295) ccw projected
  line L14 (124.0832, 122.5511) -> (124.5462, 122.2183) projected
  arc A57 (124.5462, 122.2183) -> (123.4257, 120.5415) centre (148.5, 105.0002) ccw projected
  line L15 (123.4257, 120.5415) -> (122.9411, 120.8418) projected
  arc A58 (122.9411, 120.8418) -> (122.6108, 121.0022) centre (121.5747, 118.4483) ccw projected
  arc A59 (122.6108, 121.0022) -> (121.3801, 121.3831) centre (119.769, 113.9974) ccw projected
  arc A60 (121.3801, 121.3831) -> (118.8721, 121.6791) centre (118.6096, 108.6825) ccw projected
  arc A61 (118.8721, 121.6791) -> (118.1715, 120.3685) centre (148.5, 105.0002) ccw projected
  arc A62 (118.1715, 120.3685) -> (119.811, 118.4477) centre (128.832, 127.8073) ccw projected
  arc A63 (119.811, 118.4477) -> (120.8115, 117.6359) centre (125.057, 123.8905) ccw projected
  arc A64 (120.8115, 117.6359) -> (121.1284, 117.4504) centre (122.3594, 119.9163) ccw projected
  line L16 (121.1284, 117.4504) -> (121.6473, 117.2143) projected
  arc A65 (121.6473, 117.2143) -> (120.8756, 115.3511) centre (148.5, 105.0002) ccw projected
  line L17 (120.8756, 115.3511) -> (120.3417, 115.5512) projected
  arc A66 (120.3417, 115.5512) -> (119.9864, 115.644) centre (119.4685, 112.937) ccw projected
  arc A67 (119.9864, 115.644) -> (118.705, 115.7775) centre (118.5657, 108.2194) ccw projected
  arc A68 (118.705, 115.7775) -> (116.1874, 115.5785) centre (118.4655, 102.7804) ccw projected
  arc A69 (116.1874, 115.5785) -> (115.7561, 114.1565) centre (148.5, 105.0002) ccw projected
  arc A70 (115.7561, 114.1565) -> (117.7388, 112.5923) centre (124.7605, 123.5321) ccw projected
  arc A71 (117.7388, 112.5923) -> (118.8784, 111.9914) centre (121.8221, 118.9541) ccw projected
  arc A72 (118.8784, 111.9914) -> (119.2254, 111.8712) centre (119.9517, 114.5299) ccw projected
  line L18 (119.2254, 111.8712) -> (119.7804, 111.7409) projected
  arc A73 (119.7804, 111.7409) -> (119.387, 109.763) centre (148.5, 105.0002) ccw projected
  line L19 (119.387, 109.763) -> (118.8243, 109.855) projected
  arc A74 (118.8243, 109.855) -> (118.4578, 109.8768) centre (118.4779, 107.1208) ccw projected
  arc A75 (118.4578, 109.8768) -> (117.175, 109.7577) centre (118.5129, 102.3176) ccw projected
  arc A76 (117.175, 109.7577) -> (114.7446, 109.0714) centre (119.4757, 96.9636) ccw projected
  arc A77 (114.7446, 109.0714) -> (114.5989, 107.5925) centre (148.5, 105.0002) ccw projected
  arc A78 (114.5989, 107.5925) -> (116.8487, 106.4453) centre (121.6012, 118.5446) ccw projected
  arc A79 (116.8487, 106.4453) -> (118.0837, 106.0781) centre (119.6124, 113.4813) ccw projected
  arc A80 (118.0837, 106.0781) -> (118.4474, 106.028) centre (118.641, 108.7773) ccw projected
  line L20 (118.4474, 106.028) -> (119.0172, 106.0085) projected
  arc A81 (119.0172, 106.0085) -> (119.0172, 103.9918) centre (148.5, 105.0002) ccw projected
  line L21 (119.0172, 103.9918) -> (118.4474, 103.9723) projected
  arc A82 (118.4474, 103.9723) -> (118.0837, 103.9222) centre (118.641, 101.223) ccw projected
  arc A83 (118.0837, 103.9222) -> (116.8487, 103.5551) centre (119.6124, 96.519) ccw projected
  arc A84 (116.8487, 103.5551) -> (114.5989, 102.4078) centre (121.6012, 91.4557) ccw projected
  arc A85 (114.5989, 102.4078) -> (114.7446, 100.9289) centre (148.5, 105.0002) ccw projected
  arc A86 (114.7446, 100.9289) -> (117.175, 100.2426) centre (119.4757, 113.0367) ccw projected
  arc A87 (117.175, 100.2426) -> (118.4578, 100.1235) centre (118.5129, 107.6827) ccw projected
  arc A88 (118.4578, 100.1235) -> (118.8243, 100.1453) centre (118.4779, 102.8796) ccw projected
  line L22 (118.8243, 100.1453) -> (119.387, 100.2373) projected
  arc A89 (119.387, 100.2373) -> (119.7804, 98.2594) centre (148.5, 105.0002) ccw projected
  line L23 (119.7804, 98.2594) -> (119.2254, 98.1291) projected
  arc A90 (119.2254, 98.1291) -> (118.8784, 98.009) centre (119.9517, 95.4704) ccw projected
  arc A91 (118.8784, 98.009) -> (117.7388, 97.408) centre (121.8221, 91.0463) ccw projected
  arc A92 (117.7388, 97.408) -> (115.7561, 95.8439) centre (124.7605, 86.4683) ccw projected
  arc A93 (115.7561, 95.8439) -> (116.1874, 94.4218) centre (148.5, 105.0002) ccw projected
  arc A94 (116.1874, 94.4218) -> (118.705, 94.2229) centre (118.4655, 107.2199) ccw projected
  arc A95 (118.705, 94.2229) -> (119.9864, 94.3563) centre (118.5657, 101.781) ccw projected
  arc A96 (119.9864, 94.3563) -> (120.3417, 94.4491) centre (119.4685, 97.0633) ccw projected
  line L24 (120.3417, 94.4491) -> (120.8756, 94.6492) projected
  arc A97 (120.8756, 94.6492) -> (121.6473, 92.786) centre (148.5, 105.0002) ccw projected
  line L25 (121.6473, 92.786) -> (121.1284, 92.5499) projected
  arc A98 (121.1284, 92.5499) -> (120.8115, 92.3644) centre (122.3594, 90.084) ccw projected
  arc A99 (120.8115, 92.3644) -> (119.811, 91.5526) centre (125.057, 86.1098) ccw projected
  arc A100 (119.811, 91.5526) -> (118.1715, 89.6318) centre (128.832, 82.193) ccw projected
  arc A101 (118.1715, 89.6318) -> (118.8721, 88.3212) centre (148.5, 105.0002) ccw projected
  arc A102 (118.8721, 88.3212) -> (121.3801, 88.6172) centre (118.6096, 101.3178) ccw projected
  arc A103 (121.3801, 88.6172) -> (122.6108, 88.9981) centre (119.769, 96.0029) ccw projected
  arc A104 (122.6108, 88.9981) -> (122.9411, 89.1585) centre (121.5747, 91.552) ccw projected
  line L26 (122.9411, 89.1585) -> (123.4257, 89.4588) projected
  arc A105 (123.4257, 89.4588) -> (124.5462, 87.782) centre (148.5, 105.0002) ccw projected
  line L27 (124.5462, 87.782) -> (124.0832, 87.4492) projected
  arc A106 (124.0832, 87.4492) -> (123.8086, 87.2055) centre (125.7717, 85.2708) ccw projected
  arc A107 (123.8086, 87.2055) -> (122.9858, 86.2141) centre (129.1927, 81.8993) ccw projected
  arc A108 (122.9858, 86.2141) -> (121.7525, 84.0103) centre (133.6594, 78.7942) ccw projected
  arc A109 (121.7525, 84.0103) -> (122.6952, 82.8616) centre (148.5, 105.0002) ccw projected
  arc A110 (122.6952, 82.8616) -> (125.0973, 83.6412) centre (119.9023, 95.5573) ccw projected
  arc A111 (125.0973, 83.6412) -> (126.2301, 84.2548) centre (122.0763, 90.5707) ccw projected
  arc A112 (126.2301, 84.2548) -> (126.5228, 84.4766) centre (124.7157, 86.5576) ccw projected
  line L28 (126.5228, 84.4766) -> (126.9395, 84.8657) projected
  arc A113 (126.9395, 84.8657) -> (128.3655, 83.4397) centre (148.5, 105.0002) ccw projected
  line L29 (128.3655, 83.4397) -> (127.9764, 83.023) projected
  arc A114 (127.9764, 83.023) -> (127.7546, 82.7303) centre (130.0574, 81.2159) ccw projected
  arc A115 (127.7546, 82.7303) -> (127.141, 81.5975) centre (134.0705, 78.5765) ccw projected
  arc A116 (127.141, 81.5975) -> (126.3614, 79.1954) centre (139.0571, 76.4025) ccw projected
  arc A117 (126.3614, 79.1954) -> (127.5101, 78.2527) centre (148.5, 105.0002) ccw projected
  arc A118 (127.5101, 78.2527) -> (129.7139, 79.486) centre (122.294, 90.1596) ccw projected
  arc A119 (129.7139, 79.486) -> (130.7053, 80.3088) centre (125.3991, 85.6929) ccw projected
  arc A120 (130.7053, 80.3088) -> (130.949, 80.5834) centre (128.7706, 82.2718) ccw projected
  line L30 (130.949, 80.5834) -> (131.2818, 81.0464) projected
  arc A121 (131.2818, 81.0464) -> (132.9586, 79.9259) centre (148.5, 105.0002) ccw projected
  line L31 (132.9586, 79.9259) -> (132.6583, 79.4413) projected
  arc A122 (132.6583, 79.4413) -> (132.4979, 79.111) centre (135.0518, 78.0749) ccw projected
  arc A123 (132.4979, 79.111) -> (132.117, 77.8803) centre (139.5027, 76.2692) ccw projected
  arc A124 (132.117, 77.8803) -> (131.821, 75.3722) centre (144.8176, 75.1098) ccw projected
  arc A125 (131.821, 75.3722) -> (133.1316, 74.6717) centre (148.5, 105.0002) ccw projected
  arc A126 (133.1316, 74.6717) -> (135.0525, 76.3112) centre (125.6928, 85.3322) ccw projected
  arc A127 (135.0525, 76.3112) -> (135.8642, 77.3117) centre (129.6096, 81.5572) ccw projected
  arc A128 (135.8642, 77.3117) -> (136.0497, 77.6286) centre (133.5838, 78.8596) ccw projected
  line L32 (136.0497, 77.6286) -> (136.2858, 78.1475) projected
  arc A129 (136.2858, 78.1475) -> (138.149, 77.3758) centre (148.5, 105.0002) ccw projected
  line L33 (138.149, 77.3758) -> (137.949, 76.8419) projected
  arc A130 (137.949, 76.8419) -> (137.8561, 76.4866) centre (140.5631, 75.9687) ccw projected
  arc A131 (137.8561, 76.4866) -> (137.7227, 75.2052) centre (145.2808, 75.0659) ccw projected
  arc A132 (137.7227, 75.2052) -> (137.9216, 72.6876) centre (150.7197, 74.9657) ccw projected
  arc A133 (137.9216, 72.6876) -> (139.3437, 72.2563) centre (148.5, 105.0002) ccw projected
  arc A134 (139.3437, 72.2563) -> (140.9078, 74.239) centre (129.9681, 81.2607) ccw projected
  arc A135 (140.9078, 74.239) -> (141.5088, 75.3786) centre (134.5461, 78.3223) ccw projected
  arc A136 (141.5088, 75.3786) -> (141.6289, 75.7256) centre (138.9702, 76.4519) ccw projected
  line L34 (141.6289, 75.7256) -> (141.7592, 76.2806) projected
  arc A137 (141.7592, 76.2806) -> (143.7371, 75.8872) centre (148.5, 105.0002) ccw projected
  line L35 (143.7371, 75.8872) -> (143.6451, 75.3245) projected
  arc A138 (143.6451, 75.3245) -> (143.6233, 74.958) centre (146.3794, 74.9781) ccw projected
  arc A139 (143.6233, 74.958) -> (143.7424, 73.6752) centre (151.1825, 75.0131) ccw projected
  arc A140 (143.7424, 73.6752) -> (144.4287, 71.2448) centre (156.5365, 75.9759) ccw projected
  arc A141 (144.4287, 71.2448) -> (145.9076, 71.0991) centre (148.5, 105.0002) ccw projected
  arc A142 (145.9076, 71.0991) -> (147.0549, 73.3489) centre (134.9555, 78.1014) ccw projected
  arc A143 (147.0549, 73.3489) -> (147.422, 74.5839) centre (140.0188, 76.1126) ccw projected
  arc A144 (147.422, 74.5839) -> (147.4721, 74.9476) centre (144.7228, 75.1412) ccw projected
  line L36 (147.4721, 74.9476) -> (147.4916, 75.5174) projected
  arc A145 (147.4916, 75.5174) -> (149.5083, 75.5174) centre (148.5, 105.0002) ccw projected
  line L37 (149.5083, 75.5174) -> (149.5278, 74.9476) projected
  arc A146 (149.5278, 74.9476) -> (149.5779, 74.5839) centre (152.2771, 75.1412) ccw projected
  arc A147 (149.5779, 74.5839) -> (149.9451, 73.3489) centre (156.9811, 76.1126) ccw projected
  arc A148 (149.9451, 73.3489) -> (151.0923, 71.0991) centre (162.0444, 78.1014) ccw projected
  arc A149 (151.0923, 71.0991) -> (152.5712, 71.2448) centre (148.5, 105.0002) ccw projected
  arc A150 (152.5712, 71.2448) -> (153.2575, 73.6752) centre (140.4634, 75.9759) ccw projected
  arc A151 (153.2575, 73.6752) -> (153.3766, 74.958) centre (145.8174, 75.0131) ccw projected
  arc A152 (153.3766, 74.958) -> (153.3548, 75.3245) centre (150.6206, 74.9781) ccw projected
  line L38 (153.3548, 75.3245) -> (153.2628, 75.8872) projected
  arc A153 (153.2628, 75.8872) -> (155.2407, 76.2806) centre (148.5, 105.0002) ccw projected
  line L39 (155.2407, 76.2806) -> (155.371, 75.7256) projected
  arc A154 (155.371, 75.7256) -> (155.4912, 75.3786) centre (158.0297, 76.4519) ccw projected
  arc A155 (155.4912, 75.3786) -> (156.0922, 74.239) centre (162.4539, 78.3223) ccw projected
  arc A156 (156.0922, 74.239) -> (157.6563, 72.2563) centre (167.0319, 81.2607) ccw projected
  arc A157 (157.6563, 72.2563) -> (159.0783, 72.6876) centre (148.5, 105.0002) ccw projected
  arc A158 (159.0783, 72.6876) -> (159.2773, 75.2052) centre (146.2802, 74.9657) ccw projected
  arc A159 (159.2773, 75.2052) -> (159.1439, 76.4866) centre (151.7192, 75.0659) ccw projected
  arc A160 (159.1439, 76.4866) -> (159.051, 76.8419) centre (156.4368, 75.9687) ccw projected
  line L40 (159.051, 76.8419) -> (158.8509, 77.3758) projected
  arc A161 (158.8509, 77.3758) -> (160.7141, 78.1475) centre (148.5, 105.0002) ccw projected
  line L41 (160.7141, 78.1475) -> (160.9502, 77.6286) projected
  arc A162 (160.9502, 77.6286) -> (161.1357, 77.3117) centre (163.4161, 78.8596) ccw projected
  arc A163 (161.1357, 77.3117) -> (161.9475, 76.3112) centre (167.3903, 81.5572) ccw projected
  arc A164 (161.9475, 76.3112) -> (163.8683, 74.6717) centre (171.3071, 85.3322) ccw projected
  arc A165 (163.8683, 74.6717) -> (165.1789, 75.3722) centre (148.5, 105.0002) ccw projected
  arc A166 (165.1789, 75.3722) -> (164.8829, 77.8803) centre (152.1823, 75.1098) ccw projected
  arc A167 (164.8829, 77.8803) -> (164.502, 79.111) centre (157.4972, 76.2692) ccw projected
  arc A168 (164.502, 79.111) -> (164.3416, 79.4413) centre (161.9481, 78.0749) ccw projected
  line L42 (164.3416, 79.4413) -> (164.0413, 79.9259) projected
  arc A169 (164.0413, 79.9259) -> (165.7181, 81.0464) centre (148.5, 105.0002) ccw projected
  line L43 (165.7181, 81.0464) -> (166.0509, 80.5834) projected
  arc A170 (166.0509, 80.5834) -> (166.2947, 80.3088) centre (168.2293, 82.2718) ccw projected
  arc A171 (166.2947, 80.3088) -> (167.286, 79.486) centre (171.6009, 85.6929) ccw projected
  arc A172 (167.286, 79.486) -> (169.4898, 78.2527) centre (174.7059, 90.1596) ccw projected
  arc A173 (169.4898, 78.2527) -> (170.6385, 79.1954) centre (148.5, 105.0002) ccw projected
  arc A174 (170.6385, 79.1954) -> (169.8589, 81.5975) centre (157.9429, 76.4025) ccw projected
  arc A175 (169.8589, 81.5975) -> (169.2453, 82.7303) centre (162.9294, 78.5765) ccw projected
  arc A176 (169.2453, 82.7303) -> (169.0235, 83.023) centre (166.9426, 81.2159) ccw projected
  line L44 (169.0235, 83.023) -> (168.6344, 83.4397) projected
  arc A177 (168.6344, 83.4397) -> (170.0604, 84.8657) centre (148.5, 105.0002) ccw projected
  line L45 (170.0604, 84.8657) -> (170.4771, 84.4766) projected
  arc A178 (170.4771, 84.4766) -> (170.7698, 84.2548) centre (172.2843, 86.5576) ccw projected
  arc A179 (170.7698, 84.2548) -> (171.9026, 83.6412) centre (174.9236, 90.5707) ccw projected
  arc A180 (171.9026, 83.6412) -> (174.3047, 82.8616) centre (177.0976, 95.5573) ccw projected
  arc A181 (174.3047, 82.8616) -> (175.2474, 84.0103) centre (148.5, 105.0002) ccw projected
  arc A182 (175.2474, 84.0103) -> (174.0142, 86.2141) centre (163.3405, 78.7942) ccw projected
  arc A183 (174.0142, 86.2141) -> (173.1913, 87.2055) centre (167.8072, 81.8993) ccw projected
  arc A184 (173.1913, 87.2055) -> (172.9167, 87.4492) centre (171.2283, 85.2708) ccw projected
  line L46 (172.9167, 87.4492) -> (172.4538, 87.782) projected
  arc A185 (172.4538, 87.782) -> (173.5742, 89.4588) centre (148.5, 105.0002) ccw projected
  line L47 (173.5742, 89.4588) -> (174.0588, 89.1585) projected
  arc A186 (174.0588, 89.1585) -> (174.3891, 88.9981) centre (175.4252, 91.552) ccw projected
  arc A187 (174.3891, 88.9981) -> (175.6199, 88.6172) centre (177.231, 96.0029) ccw projected
  arc A188 (175.6199, 88.6172) -> (178.1279, 88.3212) centre (178.3903, 101.3178) ccw projected
  arc A189 (178.1279, 88.3212) -> (178.8284, 89.6318) centre (148.5, 105.0002) ccw projected
  arc A190 (178.8284, 89.6318) -> (177.1889, 91.5526) centre (168.1679, 82.193) ccw projected
  arc A191 (177.1889, 91.5526) -> (176.1884, 92.3644) centre (171.943, 86.1098) ccw projected
  arc A192 (176.1884, 92.3644) -> (175.8716, 92.5499) centre (174.6406, 90.084) ccw projected
  line L48 (175.8716, 92.5499) -> (175.3526, 92.786) projected
  arc A193 (175.3526, 92.786) -> (176.1244, 94.6492) centre (148.5, 105.0002) ccw projected
  line L49 (176.1244, 94.6492) -> (176.6582, 94.4491) projected
  arc A194 (176.6582, 94.4491) -> (177.0135, 94.3563) centre (177.5315, 97.0633) ccw projected
  arc A195 (177.0135, 94.3563) -> (178.2949, 94.2229) centre (178.4342, 101.781) ccw projected
  arc A196 (178.2949, 94.2229) -> (180.8125, 94.4218) centre (178.5344, 107.2199) ccw projected
  arc A197 (180.8125, 94.4218) -> (181.2438, 95.8439) centre (148.5, 105.0002) ccw projected
  arc A198 (181.2438, 95.8439) -> (179.2611, 97.408) centre (172.2395, 86.4683) ccw projected
  arc A199 (179.2611, 97.408) -> (178.1215, 98.009) centre (175.1778, 91.0463) ccw projected
  arc A200 (178.1215, 98.009) -> (177.7745, 98.1291) centre (177.0483, 95.4704) ccw projected
  line L50 (177.7745, 98.1291) -> (177.2195, 98.2594) projected
  arc A201 (177.2195, 98.2594) -> (177.6129, 100.2373) centre (148.5, 105.0002) ccw projected
  line L51 (177.6129, 100.2373) -> (178.1756, 100.1453) projected
  arc A202 (178.1756, 100.1453) -> (178.5421, 100.1235) centre (178.522, 102.8796) ccw projected
  arc A203 (178.5421, 100.1235) -> (179.825, 100.2426) centre (178.487, 107.6827) ccw projected
  arc A204 (179.825, 100.2426) -> (182.2553, 100.9289) centre (177.5242, 113.0367) ccw projected
  arc A205 (182.2553, 100.9289) -> (182.401, 102.4078) centre (148.5, 105.0002) ccw projected
  arc A206 (182.401, 102.4078) -> (180.1512, 103.5551) centre (175.3987, 91.4557) ccw projected
  arc A207 (180.1512, 103.5551) -> (178.9163, 103.9222) centre (177.3875, 96.519) ccw projected
  arc A208 (178.9163, 103.9222) -> (178.5525, 103.9723) centre (178.3589, 101.223) ccw projected
  line L52 (178.5525, 103.9723) -> (177.9827, 103.9918) projected
  arc A209 (177.9827, 103.9918) -> (177.9827, 106.0085) centre (148.5, 105.0002) ccw projected
  line L53 (177.9827, 106.0085) -> (178.5525, 106.028) projected